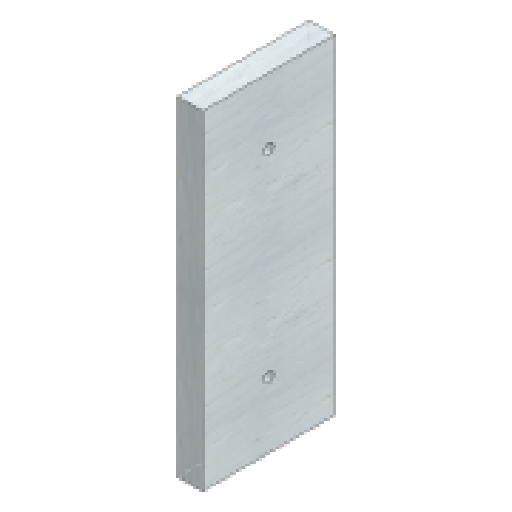
# Autodesk Inventor part: H
Saved by Autodesk Inventor 2024 (Build 280153000, 153)
## iProperties
Created: 2024-03-20
Part Number: H
Material: Generic
Document SubType Name: Modeling
Designer: marco
Density: 1 g/cm^3
Appearance: Wood - Painted White
Author: marco
Autodesk Inventor part; units mm, degrees
ref_plane "YZ Plane" through (0, 0, 0) normal (1, 0, 0) x (0, 1, 0)
ref_plane "XZ Plane" through (0, 0, 0) normal (0, 1, 0) x (-1, 0, 0)
ref_plane "XY Plane" through (0, 0, 0) normal (0, 0, 1) x (1, 0, 0)
sketch "Sketch1" plane through (0, 0, 0) normal (1, 0, 0) x (0, 1, 0)
  line L0 (125, 50) -> (-125, 50)
  line L1 (-125, 50) -> (-125, -50)
  line L2 (-125, -50) -> (125, -50)
  line L3 (125, -50) -> (125, 50)
  line L4 (125, 50) -> (-125, -50) construction
  line L5 (-125, 50) -> (125, -50) construction
  line L6 (125, 0) -> (75, 0)
  line L7 (-125, 0) -> (-75, 0)
  circle A0 centre (-75, 0) radius 4
  circle A1 centre (75, 0) radius 4
  point P0 (0, 0)
  dimension "d0" = 250
  dimension "d1" = 100
  dimension "d2" = 50
  dimension "d3" = 50
  dimension "d4" = 8
  dimension "d5" = 8
  constraints: 16 end point, 4 midpoint, 3 horizontal, 2 centre point, 2 coincident, 2 parallel, 1 perpendicular
  measures "d0" distance of L2.end L1.end
  measures "d1" distance of L1.end L0.end
  measures "d2" distance of L6.start L6.end
  measures "d3" distance of L7.start L7.end
  measures "d4" diameter of A0
  measures "d5" diameter of A1
extrude "Extrusion1" add sketch "Sketch1" along normal mid plane 19
body "Solid1"
